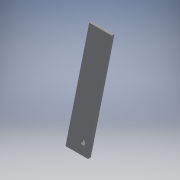
# Autodesk Inventor part: 2018 Cube Backstop Mount Angle
Saved by Autodesk Inventor 2018 (Build 220112000, 112)
## iProperties
Created: 2018-01-26
Part Number: 2018 Cube Backstop Mount Angle
Material: Generic
Document SubType Name: Modeling
Designer: Apple
Density: 1 g/cm^3
Appearance: Default
Author: Apple
Autodesk Inventor part; units mm, degrees
ref_plane "YZ Plane" through (0, 0, 0) normal (1, 0, 0) x (0, 1, 0)
ref_plane "XZ Plane" through (0, 0, 0) normal (0, 1, 0) x (-1, 0, 0)
ref_plane "XY Plane" through (0, 0, 0) normal (0, 0, 1) x (1, 0, 0)
sketch "Sketch1" plane through (0, 0, 0) normal (0, 0, 1) x (1, 0, 0)
  circle A0 centre (-641.35, -11.938) radius 2.667 projected
  line L0 (-635, -25.4) -> (-787.4, -25.4) projected
  line L1 (-611.5558, 111.1309) -> (-611.5558, 92.0809) projected
  line L2 (-611.5558, 88.9059) -> (-611.5558, 92.0809) projected
  line L3 (-655.7192, 0) -> (-787.4, 0)
  line L4 (-611.5558, 92.0809) -> (-635, -25.4)
  line L5 (-633.655, 111.1309) -> (-660.9008, -25.4)
  line L6 (-655.8321, 0) -> (-787.4, 0)
  line L7 (-633.655, 111.1309) -> (-607.7542, 111.1309)
  line L8 (-607.7542, 111.1309) -> (-611.5558, 92.0809)
  line L9 (-660.9008, -25.4) -> (-635, -25.4)
  point P0 (0, 0)
  dimension "d1" = 25.4
  constraints: 14 end point, 2 point on line, 1 collinear, 1 horizontal
  measures "d1" distance between parallel lines of L4 L5
extrude "Extrusion1" add sketch "Sketch1" along normal blind 3.175
body "Solid1"
